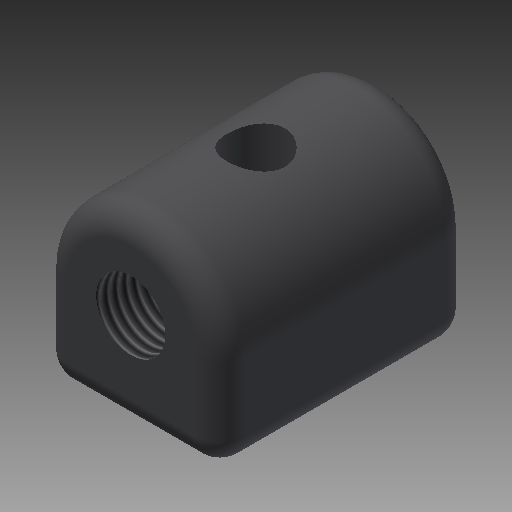
# Autodesk Inventor part: 318-03
Saved by Autodesk Inventor 2019 (Build 230136000, 136)
## iProperties
Company: Autodesk Inc.
Created: 2007-10-25
Part Number: 318-03
Document SubType Name: Modeling
Designer: Autodesk Inc.
Density: 1.32 g/cm^3
Mass: 31.5358 g
Surface Area: 67.4212 cm^2
Volume: 23.8907 cm^3
Material: Polyaryletherketone Resin
Description: BALL SCREW MOUNTING BLOCK
Appearance: Gray
Component Category: Lower Component
Author: Inventor
Autodesk Inventor part; units mm, degrees
ref_plane "YZ Plane" through (0, 0, 0) normal (1, 0, 0) x (0, 1, 0)
ref_plane "XZ Plane" through (0, 0, 0) normal (0, 1, 0) x (-1, 0, 0)
ref_plane "XY Plane" through (0, 0, 0) normal (0, 0, 1) x (1, 0, 0)
sketch "Sketch1" plane through (0, 0, 0) normal (0, 0, 1) x (1, 0, 0)
  line L0 (0, 38.6415) -> (0, -6.4403) construction
  line L1 (-24.0818, 0) -> (24.0818, 0) construction
  line L2 (-14.25, 0) -> (14.25, 0)
  line L3 (14.25, 0) -> (14.25, 15)
  line L4 (-14.25, 15) -> (-14.25, 0)
  arc A0 (0, 29.25) -> (-14.25, 15) centre (0, 15) ccw
  arc A1 (14.25, 15) -> (0, 29.25) centre (0, 15) ccw
  point P0 (0, 0)
  point P1 (-14.25, 29.25)
  dimension "d0" = 28.5
  dimension "d1" = 14.25
  dimension "d3" = 14.25
  dimension "d16" = 15
  constraints: 6 end point, 4 point on circle, 2 centre point, 2 horizontal, 2 point on line, 2 tangent, 1 concentric, 1 parallel, 1 perpendicular, 6 other
  measures "d0" distance of L2.start L2.end
  measures "d1" distance between parallel lines of L4 L0
  measures "d3" radius of A0
  measures "d16" distance from line of A0.centre L1
extrude "Extrusion1" add sketch "Sketch1" along normal mid plane 40
fillet "Fillet1" radius 4 10 edges at (14.25, 7.5, 20) (0, 29.25, 20) (-14.25, 7.5, 20) (14.25, 7.5, -20) (0, 29.25, -20) (-14.25, 7.5, -20) (14.25, 0, 0) (0, 0, 20) (-14.25, 0, 0) (0, 0, -20)
sketch "Sketch2" plane through (-10.25, 0, 16) normal (0, -1, 0) x (1, 0, 0)
  circle A0 centre (10.25, -16) radius 4.6
  dimension "d9" = 9.2
  constraints: 1 centre point, 1 coincident
  measures "d9" diameter of A0
extrude "Extrusion2" cut sketch "Sketch2" against normal up to next
fillet "Fillet2" radius 4 1 edges at (-4.6, 0, 0)
sketch "Sketch3" plane through (-10.25, 0, 16) normal (0, -1, 0) x (1, 0, 0)
  line L0 (20.5, 0) -> (20.5, -32) projected
  circle A0 centre (10.25, -16) radius 8.6 projected
  circle A1 centre (10.25, -16) radius 10.25
  circle A2 centre (10.25, -16) radius 8.6
  constraints: 2 centre point, 2 coincident, 1 concentric, 1 tangent
extrude "Extrusion3" add sketch "Sketch3" along normal blind 1.5
sketch "Sketch4" plane through (0, 0, 20) normal (0, 0, 1) x (1, 0, 0)
  line L0 (10.25, -1.5) -> (-10.25, -1.5) projected
  circle A0 centre (0, 15.675) radius 5.5
  point P0 (0, 0)
  dimension "d17" = 17.175
  dimension "d18" = 11
  constraints: 1 centre point, 1 vertical alignment
  measures "d17" distance from line of A0.centre L0
  measures "d18" diameter of A0
extrude "Extrusion4" cut sketch "Sketch4" against normal through all
thread "Thread1" size "M11x1.5" class "6H" standard "ANSI Metric M Profile" full length
equation "\"d1\" = 0.5 * d0"
body "Solid1"
